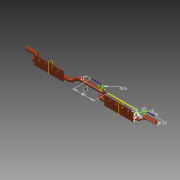
# Autodesk Inventor part: RezBorda
Saved by Autodesk Inventor 2015 (Build 190159000, 159)
## iProperties
Created: 2014-10-30
Part Number: RezBorda
Material: Copper, Wrought
Document SubType Name: Modeling
Designer: laca
Density: 8.94 g/cm^3
Appearance: Copper - Satin
Mass: 72.3578 g
Surface Area: 107.956 cm^2
Volume: 8.09371 cm^3
Author: laca
Autodesk Inventor part; units mm, degrees
ref_plane "YZ Plane" through (0, 0, 0) normal (1, 0, 0) x (0, 1, 0)
ref_plane "XZ Plane" through (0, 0, 0) normal (0, 1, 0) x (-1, 0, 0)
ref_plane "XY Plane" through (0, 0, 0) normal (0, 0, 1) x (1, 0, 0)
sketch "Sketch1" plane through (0, 0, 0) normal (0, 0, 1) x (1, 0, 0)
  line L0 (0, 0) -> (-56, 0)
  line L1 (-56, 0) -> (-56, 18)
  line L2 (-56, 18) -> (0, 18)
  line L3 (0, 18) -> (0, 0)
  circle A0 centre (-10, 13.5) radius 2
  circle A1 centre (-22, 13.5) radius 2
  circle A2 centre (-34, 13.5) radius 2
  circle A3 centre (-46, 13.5) radius 2
  dimension "d0" = 18
  dimension "d2" = 4
  dimension "d3" = 13.5
  dimension "d4" = 10
  dimension "d7" = 12
  dimension "d12" = 10
  constraints: 8 end point, 4 centre point, 2 horizontal, 2 parallel, 1 perpendicular, 6 other
  measures "d0" distance of L2.end L0.start
  measures "d2" diameter of A0
  measures "d3" distance from line of L0 A0.centre
  measures "d4" distance from line of L3 A0.centre
  measures "d7" distance of A0.centre A1.centre
  measures "d12" distance from line of L1 A3.centre
extrude "Extrusion1" add sketch "Sketch1" along normal blind 1
sketch "Sketch2" plane through (0, 0, 0) normal (1, 0, 0) x (0, 0, -1)
  circle A0 centre (2.5, 6) radius 3
  circle A1 centre (2.5, 6) radius 1.5
  line L0 (0, 18) -> (0, 0) projected
  dimension "d15" = 6
  dimension "d17" = 1.5
  dimension "d18" = 6
  dimension "d23" = 2.5
  constraints: 2 centre point, 1 coincident
  measures "d15" diameter of A0
  measures "d17" radial gap between concentric circles of A0 A1
  measures "d18" vertical distance of L0.end A0.centre
  measures "d23" distance from line of L0 A0.centre
extrude "Extrusion2" add sketch "Sketch2" against normal up to surface (56 mm away)
ref_plane "Work Plane1" through (-28, 0, 1) normal (1, 0, 0) x (0, 0, -1)
fillet "Fillet1" radius 1.5 2 edges at (-28, 4.3417, 0) (-28, 7.6583, 0)
sketch "Sketch3" plane through (-56, 0, 1) normal (-1, 0, 0) x (0, 0, 1)
  circle A0 centre (-3.5, 6) radius 1.5 projected
  circle A1 centre (-3.5, 6) radius 1.5
  arc A2 (-2.8333, 8.925) -> (-2.8333, 3.075) centre (-3.5, 6) ccw projected
  circle A3 centre (-3.5, 6) radius 3
  point P0 (-1, 0)
  constraints: 2 centre point, 2 coincident
ref_plane "Work Plane2" through (-96, 6, -2.5) normal (-1, 0, 0) x (0, 0, 1)
sketch "Sketch4" plane through (-56, 18, 0) normal (0, 1, 0) x (1, 0, 0)
  line L0 (56, 0) -> (58.461, 0)
  line L1 (64.461, 6) -> (64.461, 6)
  line L2 (70.461, 12) -> (85.461, 12)
  arc A0 (58.461, 0) -> (64.461, 6) centre (58.461, 6) ccw
  arc A1 (70.461, 12) -> (64.461, 6) centre (70.461, 6) ccw
  line L3 (0, 1.8333) -> (-8.0941, 1.8333)
  line L4 (-14.0941, 7.8333) -> (-14.0941, 7.8333)
  line L5 (56, 5.5) -> (0, 5.5) projected
  line L6 (-20.0941, 13.8333) -> (-40, 13.8333)
  arc A2 (-14.0941, 7.8333) -> (-20.0941, 13.8333) centre (-20.0941, 7.8333) ccw
  arc A3 (-14.0941, 7.8333) -> (-8.0941, 1.8333) centre (-8.0941, 7.8333) ccw
  dimension "d28" = 6
  dimension "d29" = 6
  dimension "d32" = 6
  dimension "d35" = 40
  dimension "d36" = 12
  dimension "d37" = 12
  dimension "d38" = 15
  constraints: 12 end point, 8 point on circle, 8 tangent, 4 centre point, 4 perpendicular, 2 equal radius, 2 horizontal
  measures "d28" radius of A0
  measures "d29" radius of A1
  measures "d32" radius of A2
  measures "d35" horizontal distance of L3.start L6.end
  measures "d36" distance between parallel lines of L3 L6
  measures "d37" distance between parallel lines of L0 L2
  measures "d38" distance of L2.start L2.end
sweep "Sweep1" add profiles "Sketch2" path "Sketch4" path curves L0 A0 A1 L2
sweep "Sweep2" add profiles "Sketch3" path "Sketch4" path curves L3 A3 A2 L6
mirror "Mirror4" about plane through (-96, 6, -14.5) normal (-1, 0, 0) of "Extrusion1", "Extrusion2", "Fillet1", "Sweep1", "Sweep2"
ref_plane "Work Plane4" through (-96, 6, -2.5) normal (-1, 0, 0) x (0, 0, 1)
ref_plane "Work Plane5" through (-164, 0, 1) normal (1, 0, 0) x (0, 0, -1)
equation "\"d32\" = d28"
equation "\"d37\" = d36"
body "Solid1"
